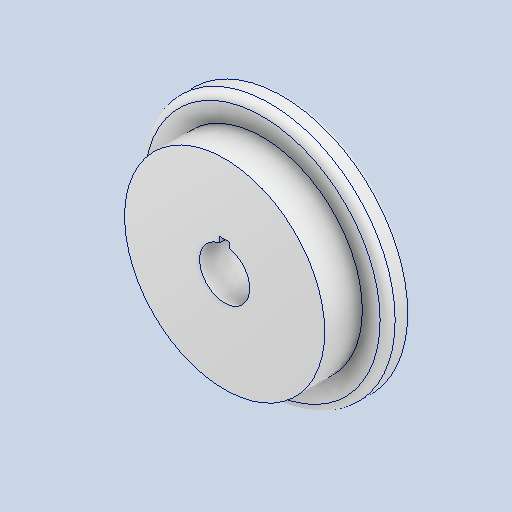
# Autodesk Inventor part: P204
Saved by Autodesk Inventor 2023 (Build 270158000, 158)
## iProperties
Created: 2022-08-23
Part Number: P204
Material: Aluminum 6061
Document SubType Name: Modeling
Designer: D.C. Eksteen
Density: 2.7 g/cm^3
Appearance: Aluminum - Flat
Author: D.C. Eksteen
Title: POWER ROLLER END CAP
Autodesk Inventor part; units mm, degrees
ref_plane "YZ Plane" through (0, 0, 0) normal (1, 0, 0) x (0, 1, 0)
ref_plane "XZ Plane" through (0, 0, 0) normal (0, 1, 0) x (-1, 0, 0)
ref_plane "XY Plane" through (0, 0, 0) normal (0, 0, 1) x (1, 0, 0)
sketch "Sketch1" plane through (0, 0, 0) normal (0, 0, 1) x (1, 0, 0)
  circle A0 centre (0, 0) radius 50
  dimension "d0" = 100
  constraints: 1 centre point, 1 coincident
  measures "d0" diameter of A0
extrude "Extrusion1" add sketch "Sketch1" along normal blind 10
sketch "Sketch2" plane through (0, 0, 10) normal (0, 0, 1) x (1, 0, 0)
  circle A0 centre (0, 0) radius 39.9
  dimension "d3" = 79.8
  constraints: 1 centre point, 1 coincident
  measures "d3" diameter of A0
extrude "Extrusion2" add sketch "Sketch2" along normal blind 15
fillet "Fillet1" radius 3 1 edges at (-50, 0, 10)
sketch "Sketch3" plane through (0, 0, 0) normal (0, 0, -1) x (-1, 0, 0)
  point P0 (0, 0)
  point P1 (0, 0)
  constraints: 1 coincident
hole "Hole1" at (0, 0, 0) direction (0, 0, 1) diameter 20 end through all
fillet "Fillet2" radius 2 1 edges at (-50, 0, 0)
sketch "Sketch5" plane through (0, 0, 0) normal (0, 0, -1) x (-1, 0, 0)
  circle A0 centre (0, 0) radius 10 projected
  line L0 (-2, 12) -> (2, 12)
  line L1 (2, 12) -> (2, 8)
  line L2 (2, 8) -> (-2, 8)
  line L3 (-2, 8) -> (-2, 12)
  point P0 (-2, 10)
  point P1 (-2, 9.798)
  point P2 (2, 9.798)
  dimension "d19" = 4
  dimension "d20" = 4
  dimension "d21" = 2
  dimension "d22" = 12
  constraints: 8 end point, 2 parallel, 1 horizontal, 1 midpoint, 1 perpendicular
  measures "d19" distance of L1.end L2.end
  measures "d20" distance of L0.end L1.end
  measures "d21" horizontal distance of point (0, 0) point (-2, 10)
  measures "d22" distance from line of point (0, 0) L0
extrude "Extrusion4" cut sketch "Sketch5" against normal through all contours A0 L3 L0 L1
body "Solid1"
